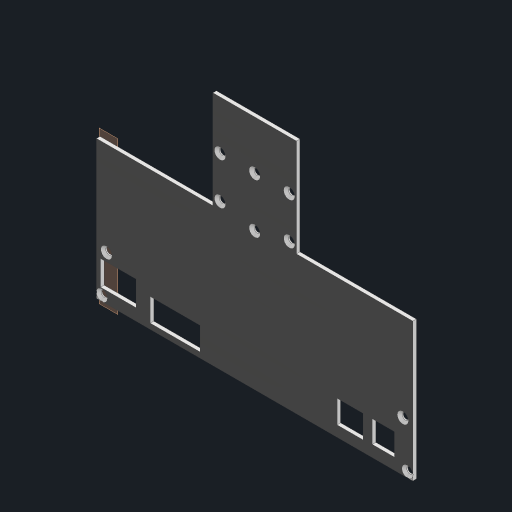
# Autodesk Inventor part: ceil
Saved by Autodesk Inventor 2023 (Build 270158000, 158)
## iProperties
Created: 2024-04-25
Part Number: ceil
Material: Generic
Document SubType Name: Modeling
Designer: szymo
Density: 1 g/cm^3
Appearance: Default
Author: szymo
Autodesk Inventor part; units mm, degrees
ref_plane "YZ Plane" through (0, 0, 0) normal (1, 0, 0) x (0, 1, 0)
ref_plane "XZ Plane" through (0, 0, 0) normal (0, 1, 0) x (-1, 0, 0)
ref_plane "XY Plane" through (0, 0, 0) normal (0, 0, 1) x (1, 0, 0)
ref_plane "Work Plane1" through (0, 0, 0) normal (0, 0, 1) x (1, 0, 0)
sketch "Sketch1" plane through (0, 0, 0) normal (0, 0, 1) x (1, 0, 0)
  circle A0 centre (3, -74.8889) radius 2.3 projected
  line L0 (3, 0) -> (3, -44.7889) projected
  line L1 (0, 0) -> (3, 0) projected
  line L2 (0, -77.8889) -> (0, 0) projected
  line L3 (0, -77.8889) -> (6, -77.8889) projected
  line L4 (6, -71.8889) -> (6, -77.8889) projected
  line L5 (6, -71.8889) -> (1.6, -71.8889) projected
  line L6 (1.6, -71.8889) -> (1.6, -56.7889) projected
  line L7 (1.6, -56.7889) -> (9.6, -56.7889) projected
  line L8 (9.6, -44.7889) -> (9.6, -56.7889) projected
  line L9 (3, -44.7889) -> (9.6, -44.7889) projected
  circle A1 centre (5.6, -52.7889) radius 2.6 projected
  circle A2 centre (172.4, -49.8889) radius 2.6 projected
  circle A3 centre (175, -74.8889) radius 2.3 projected
  line L10 (168.4, -41.8889) -> (175, -41.8889) projected
  line L11 (168.4, -53.8889) -> (168.4, -41.8889) projected
  line L12 (175, -53.8889) -> (168.4, -53.8889) projected
  line L13 (175, -53.8889) -> (175, -71.8889) projected
  line L14 (175, -71.8889) -> (172, -71.8889) projected
  line L15 (172, -71.8889) -> (172, -77.8889) projected
  line L16 (178, -77.8889) -> (172, -77.8889) projected
  line L17 (178, -77.8889) -> (178, 0) projected
  line L18 (178, 0) -> (175, 0) projected
  line L19 (175, 0) -> (175, -41.8889) projected
  line L20 (65.5, 41.9823) -> (65.5, 55) projected
  line L21 (112.5, 41.9823) -> (112.5, 55) projected
  line L22 (62.4925, 0) -> (3, 0) projected
  line L23 (115.5075, 0) -> (175, 0) projected
  line L24 (65.5, 55) -> (112.5, 55)
  line L25 (112.5, 55) -> (112.5, 0)
  line L26 (112.5, 0) -> (65.5, 0)
  line L27 (65.5, 0) -> (65.5, 55)
  line L28 (178, 0) -> (0, 0)
  line L29 (0, 0) -> (0, -77.8889)
  line L30 (0, -77.8889) -> (178, -77.8889)
  line L31 (178, -77.8889) -> (178, 0)
  line L32 (31.25, -62.8889) -> (31.25, -73.8889) projected
  line L33 (31.25, -73.8889) -> (57.25, -73.8889) projected
  line L34 (57.25, -73.8889) -> (57.25, -62.8889) projected
  line L35 (57.25, -62.8889) -> (31.25, -62.8889) projected
  line L36 (21.2501, -70.339) -> (21.2501, -58.3388) projected
  line L37 (21.2501, -58.3388) -> (3.2499, -58.3388) projected
  line L38 (3.2499, -70.339) -> (21.2501, -70.339) projected
  line L39 (3.2499, -58.3388) -> (3.2499, -70.339) projected
  line L40 (156.2, -70.4889) -> (156.2, -59.9889) projected
  line L41 (166.7, -59.9889) -> (156.2, -59.9889) projected
  line L42 (166.7, -59.9889) -> (166.7, -70.4889) projected
  line L43 (156.2, -70.4889) -> (166.7, -70.4889) projected
  line L44 (149, -59.8889) -> (149, -70.8889) projected
  line L45 (149, -70.8889) -> (136.35, -70.8889) projected
  line L46 (136.35, -70.8889) -> (136.35, -59.8889) projected
  line L47 (136.35, -59.8889) -> (149, -59.8889) projected
  line L48 (135, -53.8889) -> (135, -71.8889) projected
  line L49 (135, -71.8889) -> (175, -71.8889) projected
  line L50 (175, -71.8889) -> (175, -53.8889) projected
  line L51 (175, -53.8889) -> (135, -53.8889) projected
  circle A4 centre (137.85, -56.7389) radius 1.5 projected
  circle A5 centre (172.15, -56.7389) radius 1.5 projected
  line L52 (2.2499, -57.3388) -> (22.2501, -57.3388)
  line L53 (22.2501, -57.3388) -> (22.2501, -71.339)
  line L54 (22.2501, -71.339) -> (2.2499, -71.339)
  line L55 (2.2499, -71.339) -> (2.2499, -57.3388)
  line L56 (30.25, -61.8889) -> (30.25, -74.8889)
  line L57 (30.25, -74.8889) -> (58.25, -74.8889)
  line L58 (58.25, -74.8889) -> (58.25, -61.8889)
  line L59 (58.25, -61.8889) -> (30.25, -61.8889)
  line L60 (155.2, -58.9889) -> (155.2, -71.4889)
  line L61 (155.2, -71.4889) -> (167.7, -71.4889)
  line L62 (167.7, -71.4889) -> (167.7, -58.9889)
  line L63 (167.7, -58.9889) -> (155.2, -58.9889)
  line L64 (150, -58.8889) -> (150, -71.8889)
  line L65 (150, -71.8889) -> (135.35, -71.8889)
  line L66 (135.35, -71.8889) -> (135.35, -58.8889)
  line L67 (135.35, -58.8889) -> (150, -58.8889)
  dimension "d0" = 1
  dimension "d1" = 1
  dimension "d2" = 1
  dimension "d3" = 1
  constraints: 48 end point, 4 parallel, 3 perpendicular, 2 horizontal, 12 other
  measures "d0" distance between parallel lines of L37 L52
  measures "d1" distance between parallel lines of L35 L59
  measures "d2" distance between parallel lines of L41 L63
  measures "d3" distance between parallel lines of L47 L67
extrude "Extrusion1" add sketch "Sketch1" along normal blind 2 contours A0 | L22 L28 L26 L23 L19 L10 L11 L51 L48 L49 L15 L30 L4 L5 L6 L7 L8 L9 L0 | L0 L9 L8 L7 L6 L5 L4 L3 L2 L1 | L27 L20 L24 L21 L25 L26 | L15 L14 L13 L12 L11 L10 L19 L18 L17 L16 | L49 L64 L67 L66 L48 L51 L12 L13 L14 | A1 | A2 | A3 | A4 | A5
sketch "Sketch2" plane through (0, 0, 2) normal (0, 0, 1) x (1, 0, 0)
  circle A0 centre (3, -74.8889) radius 2 projected
  circle A1 centre (5.6, -52.7889) radius 2.6 projected
  circle A2 centre (172.4, -49.8889) radius 2.6 projected
  circle A3 centre (175, -74.8889) radius 2 projected
  circle A4 centre (108.4457, 27.5) radius 2.3 projected
  circle A5 centre (69.5, 27.5) radius 2.3 projected
  circle A6 centre (69.5, 4.0875) radius 2.3 projected
  circle A7 centre (108.4841, 4.0875) radius 2.3 projected
  circle A8 centre (89, -0.5003) radius 2.3 projected
  circle A9 centre (89, 27.5) radius 2.3 projected
  point P0 (0, 0)
  constraints: 10 coincident
hole "Hole1" at (3, -74.8889, 2) at (5.6, -52.7889, 2) at (175, -74.8889, 2) at (172.4, -49.8889, 2) at (89, -0.5003, 2) at (69.5, 4.0875, 2) at (108.4841, 4.0875, 2) at (89, 27.5, 2) at (69.5, 27.5, 2) at (108.4457, 27.5, 2) direction (0, 0, -1) diameter 3.6 end through all countersink diameter 6.3 countersink angle 90 clearance for "Countersunk Flat Head Screw ISO 2009/7046" size "M3" standard "ISO"
body "Solid1"
